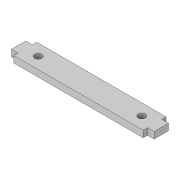
# Autodesk Inventor part: camera_mount
Saved by Autodesk Inventor 2017 (Build 210142000, 142)
## iProperties
Created: 2019-06-13
Part Number: camera_mount
Material: Generic
Document SubType Name: Modeling
Designer: markg
Density: 1 g/cm^3
Appearance: Default
Author: markg
Autodesk Inventor part; units mm, degrees
ref_plane "YZ Plane" through (0, 0, 0) normal (1, 0, 0) x (0, 1, 0)
ref_plane "XZ Plane" through (0, 0, 0) normal (0, 1, 0) x (-1, 0, 0)
ref_plane "XY Plane" through (0, 0, 0) normal (0, 0, 1) x (1, 0, 0)
sketch "Sketch1" plane through (0, 0, 0) normal (0, 1, 0) x (-1, 0, 0)
  line L0 (0, 0) -> (-57.15, 0)
  line L1 (-57.15, 0) -> (-57.15, -10.16)
  line L2 (-57.15, -10.16) -> (0, -10.16)
  line L3 (0, -10.16) -> (0, 0)
  line L4 (0, -1.905) -> (2.921, -1.905)
  line L5 (2.921, -1.905) -> (2.921, -8.255)
  line L6 (2.921, -8.255) -> (0, -8.255)
  line L7 (0, -8.255) -> (0, -1.905)
  line L8 (-60.071, -1.905) -> (-57.15, -1.905)
  line L9 (-57.15, -1.905) -> (-57.15, -8.255)
  line L10 (-57.15, -8.255) -> (-60.071, -8.255)
  line L11 (-60.071, -8.255) -> (-60.071, -1.905)
  dimension "d0" = 57.15
  dimension "d1" = 10.16
  dimension "d2" = 2.921
  dimension "d3" = 6.35
  dimension "d4" = 1.905
  dimension "d7" = 60.071
  constraints: 24 end point, 4 parallel, 3 horizontal, 2 perpendicular, 1 collinear, 1 point on line, 7 other
  measures "d0" distance of L1.end L2.end
  measures "d1" distance of L2.end L0.start
  measures "d2" distance of L5.end L6.end
  measures "d3" distance of L4.end L5.end
  measures "d4" distance from line of L0.start L4
  measures "d7" distance of L4.start L8.start
extrude "Extrusion1" add sketch "Sketch1" along normal blind 2.921
sketch "Sketch2" plane through (0, 2.921, 0) normal (0, 1, 0) x (1, 0, 0)
  circle A0 centre (5.715, 5.08) radius 1.5875
  circle A1 centre (51.435, 5.08) radius 1.5875
  line L0 (0, 0) -> (57.15, 0) projected
  line L1 (0, 1.905) -> (0, 0) projected
  dimension "d14" = 3.175
  dimension "d15" = 3.175
  dimension "d16" = 5.08
  dimension "d17" = 5.08
  dimension "d18" = 45.72
  dimension "d19" = 5.715
  constraints: 2 centre point
  measures "d14" diameter of A0
  measures "d15" diameter of A1
  measures "d16" distance from line of L0 A0.centre
  measures "d17" distance from line of L0 A1.centre
  measures "d18" distance of A1.centre A0.centre
  measures "d19" distance from line of A0.centre L1
extrude "Extrusion2" cut sketch "Sketch2" against normal blind 2.921
body "Solid1"
